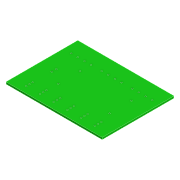
# Autodesk Inventor part: placa
Saved by Autodesk Inventor 2022 (Build 260153000, 153)
## iProperties
Created: 2022-11-21
Part Number: placa
Material: Generic
Document SubType Name: Modeling
Designer: ferna
Density: 1 g/cm^3
Appearance: Dark Green
Author: ferna
Autodesk Inventor part; units mm, degrees
ref_plane "YZ Plane" through (0, 0, 0) normal (1, 0, 0) x (0, 1, 0)
ref_plane "XZ Plane" through (0, 0, 0) normal (0, 1, 0) x (-1, 0, 0)
ref_plane "XY Plane" through (0, 0, 0) normal (0, 0, 1) x (1, 0, 0)
sketch "Sketch1" plane through (0, 0, 0) normal (0, 1, 0) x (-1, 0, 0)
  line L0 (0, 0) -> (75, 0)
  line L1 (75, 0) -> (75, -56)
  line L2 (75, -56) -> (0, -56)
  line L3 (0, -56) -> (0, 0)
  dimension "d0" = 75
  dimension "d1" = 56
  constraints: 8 end point, 2 parallel, 1 horizontal, 1 perpendicular
  measures "d0" distance of L1.end L2.end
  measures "d1" distance of L0.end L1.end
extrude "Extrusion1" add sketch "Sketch1" along normal blind 1.524
sketch "Sketch2" plane through (0, 1.524, 0) normal (0, 1, 0) x (1, 0, 0)
  circle A0 centre (-64.2857, 10.08) radius 0.508
  circle A1 centre (-64.2857, 7.54) radius 0.508
  circle A2 centre (-64.2857, 5) radius 0.508
  line L0 (-75, 0) -> (0, 0) projected
  line L1 (-75, 56) -> (-75, 0) projected
  line L2 (-75, 0) -> (-64.2857, 0)
  line L3 (-64.2857, 0) -> (-64.2857, 5)
  circle A3 centre (-53.5714, 10.08) radius 0.508
  circle A4 centre (-53.5714, 7.54) radius 0.508
  circle A5 centre (-53.5714, 5) radius 0.508
  circle A6 centre (-42.8571, 10.08) radius 0.508
  circle A7 centre (-42.8571, 7.54) radius 0.508
  circle A8 centre (-42.8571, 5) radius 0.508
  circle A9 centre (-32.1429, 10.08) radius 0.508
  circle A10 centre (-32.1429, 7.54) radius 0.508
  circle A11 centre (-32.1429, 5) radius 0.508
  circle A12 centre (-21.4286, 10.08) radius 0.508
  circle A13 centre (-21.4286, 7.54) radius 0.508
  circle A14 centre (-21.4286, 5) radius 0.508
  circle A15 centre (-10.7143, 10.08) radius 0.508
  circle A16 centre (-10.7143, 7.54) radius 0.508
  circle A17 centre (-10.7143, 5) radius 0.508
  dimension "d6" = 10.7143
  dimension "d7" = 5
  dimension "d10" = 10.7143
  constraints: 18 centre point, 4 end point, 1 horizontal, 1 perpendicular, 1 point on line, 30 other
  measures "d6" distance of L0.start L2.end
  measures "d7" distance of L2.end L3.end
  measures "d10" distance of A0.centre A3.centre
extrude "Extrusion2" cut sketch "Sketch2" against normal through all
sketch "Sketch3" plane through (0, 1.524, 0) normal (0, 1, 0) x (1, 0, 0)
  circle A0 centre (-53.3171, 36.0669) radius 0.51
  circle A1 centre (-13.3171, 36.0669) radius 0.51
  circle A2 centre (-13.3171, 19.0669) radius 0.51
  circle A3 centre (-53.3171, 19.0669) radius 0.51
  point P0 (0, 0)
  dimension "d17" = 1.02
  dimension "d18" = 1.02
  dimension "d19" = 1.02
  dimension "d20" = 1.02
  constraints: 4 centre point, 1 coincident
  measures "d17" diameter of A0
  measures "d18" diameter of A1
  measures "d19" diameter of A2
  measures "d20" diameter of A3
extrude "Extrusion3" cut sketch "Sketch3" against normal blind 10
sketch "Sketch4" plane through (0, 1.524, 0) normal (0, 1, 0) x (1, 0, 0)
  circle A0 centre (-63.9477, 28.149) radius 0.55
  circle A1 centre (-63.9477, 24.649) radius 0.55
  point P0 (0, 0)
  constraints: 2 centre point
extrude "Extrusion4" cut sketch "Sketch4" against normal blind 10
sketch "Sketch5" plane through (0, 1.524, 0) normal (0, 1, 0) x (1, 0, 0)
  line L0 (0, 0) -> (0, 56) projected
  line L1 (0, 56) -> (0, 45)
  line L2 (0, 45) -> (-5.26, 45)
  arc A0 (-6.06, 44.6) -> (-5.26, 44.6) centre (-5.66, 44.6) ccw
  arc A1 (-29.06, 44.6) -> (-29.86, 44.6) centre (-29.46, 44.6) ccw
  arc A2 (-34.94, 44.6) -> (-34.14, 44.6) centre (-34.54, 44.6) ccw
  arc A3 (-40.26, 44.6) -> (-39.86, 44.2) centre (-39.86, 44.6) ccw
  arc A4 (-68.74, 45) -> (-69.14, 44.6) centre (-68.74, 44.6) ccw
  circle A5 centre (-5.66, 44.6) radius 0.51
  circle A6 centre (-10.74, 44.6) radius 0.51
  circle A7 centre (-16.06, 44.6) radius 0.51
  circle A8 centre (-21.14, 44.6) radius 0.51
  circle A9 centre (-29.46, 44.6) radius 0.51
  circle A10 centre (-34.54, 44.6) radius 0.51
  circle A11 centre (-39.86, 44.6) radius 0.51
  circle A12 centre (-44.94, 44.6) radius 0.51
  circle A13 centre (-53.26, 44.6) radius 0.51
  circle A14 centre (-58.34, 44.6) radius 0.51
  circle A15 centre (-63.66, 44.6) radius 0.51
  circle A16 centre (-68.74, 44.6) radius 0.51
  line L3 (-5.26, 44.2) -> (-5.26, 44.2836)
  line L4 (-5.26, 44.9164) -> (-5.26, 45)
  line L5 (-5.26, 45) -> (-5.3436, 45)
  line L6 (-5.9764, 45) -> (-6.06, 45)
  line L7 (-6.06, 45) -> (-6.06, 44.9164)
  line L8 (-6.06, 44.2836) -> (-6.06, 44.2)
  line L9 (-6.06, 44.2) -> (-5.9764, 44.2)
  line L10 (-5.3436, 44.2) -> (-5.26, 44.2)
  line L11 (-10.34, 45) -> (-10.74, 45)
  line L12 (-11.0564, 45) -> (-11.14, 45)
  line L13 (-11.14, 45) -> (-11.14, 44.9164)
  line L14 (-11.14, 44.6) -> (-11.14, 44.2)
  line L15 (-10.34, 44.2) -> (-10.34, 44.2836)
  line L16 (-10.34, 44.9164) -> (-10.34, 45)
  line L17 (-16.46, 45) -> (-16.46, 44.6)
  line L18 (-16.46, 44.2836) -> (-16.46, 44.2)
  line L19 (-16.46, 44.2) -> (-16.3764, 44.2)
  line L20 (-15.7436, 44.2) -> (-15.66, 44.2)
  line L21 (-15.66, 44.2) -> (-15.66, 44.2836)
  line L22 (-15.66, 44.9164) -> (-15.66, 45)
  line L23 (-21.54, 45) -> (-21.54, 44.9164)
  line L24 (-21.54, 44.2836) -> (-21.54, 44.2)
  line L25 (-20.74, 45) -> (-20.8236, 45)
  line L26 (-21.14, 45) -> (-21.54, 45)
  line L27 (-20.74, 44.2) -> (-20.74, 44.6)
  line L28 (-20.74, 44.9164) -> (-20.74, 45)
  line L29 (-29.86, 45) -> (-29.86, 44.9164)
  line L30 (-29.86, 44.2836) -> (-29.86, 44.2)
  line L31 (-29.06, 45) -> (-29.1436, 45)
  line L32 (-29.7764, 45) -> (-29.86, 45)
  line L33 (-29.06, 44.2) -> (-29.06, 44.6)
  line L34 (-29.06, 44.9164) -> (-29.06, 45)
  line L35 (-34.94, 45) -> (-34.94, 44.9164)
  line L36 (-34.94, 44.2836) -> (-34.94, 44.2)
  line L37 (-34.14, 45) -> (-34.54, 45)
  line L38 (-34.8564, 45) -> (-34.94, 45)
  line L39 (-34.14, 44.2) -> (-34.14, 44.6)
  line L40 (-34.14, 44.9164) -> (-34.14, 45)
  line L41 (-40.26, 45) -> (-40.26, 44.9164)
  line L42 (-40.26, 44.2836) -> (-40.26, 44.2)
  line L43 (-39.46, 44.2) -> (-39.46, 44.2836)
  line L44 (-39.46, 44.6) -> (-39.46, 45)
  line L45 (-40.26, 44.2) -> (-40.1764, 44.2)
  line L46 (-39.5436, 44.2) -> (-39.46, 44.2)
  line L47 (-45.34, 45) -> (-45.34, 44.9164)
  line L48 (-45.34, 44.2836) -> (-45.34, 44.2)
  line L49 (-44.54, 44.2) -> (-44.54, 44.2836)
  line L50 (-44.54, 44.6) -> (-44.54, 45)
  line L51 (-45.34, 44.2) -> (-45.2564, 44.2)
  line L52 (-44.6236, 44.2) -> (-44.54, 44.2)
  line L53 (-44.54, 45) -> (-44.6236, 45)
  line L54 (-45.2564, 45) -> (-45.34, 45)
  line L55 (-52.86, 44.2) -> (-52.86, 44.6)
  line L56 (-52.86, 44.9164) -> (-52.86, 45)
  line L57 (-52.86, 45) -> (-52.9436, 45)
  line L58 (-53.5764, 45) -> (-53.66, 45)
  line L59 (-53.66, 45) -> (-53.66, 44.9164)
  line L60 (-53.66, 44.2836) -> (-53.66, 44.2)
  line L61 (-53.66, 44.2) -> (-53.5764, 44.2)
  line L62 (-53.26, 44.2) -> (-52.86, 44.2)
  line L63 (-58.74, 45) -> (-58.74, 44.6)
  line L64 (-58.74, 44.2836) -> (-58.74, 44.2)
  line L65 (-58.74, 44.2) -> (-58.6564, 44.2)
  line L66 (-58.0236, 44.2) -> (-57.94, 44.2)
  line L67 (-57.94, 44.2) -> (-57.94, 44.2836)
  line L68 (-57.94, 44.9164) -> (-57.94, 45)
  line L69 (-57.94, 45) -> (-58.0236, 45)
  line L70 (-58.6564, 45) -> (-58.74, 45)
  line L71 (-64.06, 45) -> (-64.06, 44.6)
  line L72 (-64.06, 44.2836) -> (-64.06, 44.2)
  line L73 (-64.06, 44.2) -> (-63.9764, 44.2)
  line L74 (-63.3436, 44.2) -> (-63.26, 44.2)
  line L75 (-63.26, 44.2) -> (-63.26, 44.2836)
  line L76 (-63.26, 44.9164) -> (-63.26, 45)
  line L77 (-63.26, 45) -> (-63.3436, 45)
  line L78 (-63.66, 45) -> (-64.06, 45)
  line L79 (-69.14, 45) -> (-69.14, 44.6)
  line L80 (-69.14, 44.2836) -> (-69.14, 44.2)
  line L81 (-69.14, 44.2) -> (-69.0564, 44.2)
  line L82 (-68.4236, 44.2) -> (-68.34, 44.2)
  line L83 (-68.34, 44.2) -> (-68.34, 44.2836)
  line L84 (-68.34, 44.9164) -> (-68.34, 45)
  line L85 (-68.34, 45) -> (-68.4236, 45)
  line L86 (-69.0564, 45) -> (-69.14, 45)
  point P0 (5.46, 11.6)
  point P1 (5.86, 11.2)
  point P2 (-65.4628, 43.85)
  dimension "d28" = 1.02
  dimension "d35" = 1.02
  dimension "d37" = 1.02
  dimension "d39" = 1.02
  dimension "d26" = 11
  dimension "d27" = 5.26
  dimension "d29" = 1.02
  dimension "d30" = 1.02
  dimension "d31" = 1.02
  dimension "d32" = 1.02
  dimension "d33" = 1.02
  dimension "d34" = 1.02
  dimension "d36" = 1.02
  dimension "d38" = 1.02
  constraints: 172 end point, 49 point on circle, 30 tangent, 13 centre point, 1 coincident, 1 horizontal, 1 point on line, 37 other
  measures "d26" distance of L0.end L1.end
  measures "d27" distance of L1.end L2.end
  measures "d29" diameter of A6
  measures "d30" diameter of A7
  measures "d31" diameter of A8
  measures "d32" diameter of A9
  measures "d33" diameter of A10
  measures "d34" diameter of A11
  measures "d36" diameter of A13
  measures "d38" diameter of A15
extrude "Extrusion5" cut sketch "Sketch5" against normal through all contours A5 | A6 | A7 | A8 | A9 | A10 | A11 | A12 | A13 | A14 | A15 | A16
body "Solid1"
